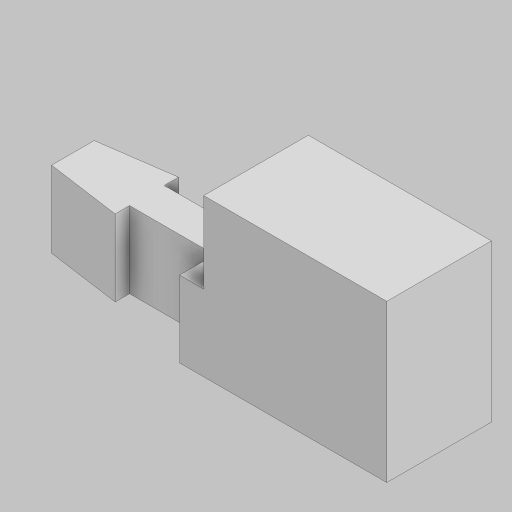
# Autodesk Inventor part: Tenon_Macho_Parametrizado
Saved by Autodesk Inventor 2023 (Build 270158000, 158)
## iProperties
Created: 2026-02-15
Part Number: Tenon_Macho_Parametrizado
Material: Genérico
Document SubType Name: Modeling
Designer: MARTIN MAESTRE
Density: 1 g/cm^3
Appearance: Valor por defecto
Author: MARTIN MAESTRE
Autodesk Inventor part; units mm, degrees
ref_plane "YZ Plane" through (0, 0, 0) normal (1, 0, 0) x (0, 1, 0)
ref_plane "XZ Plane" through (0, 0, 0) normal (0, 1, 0) x (-1, 0, 0)
ref_plane "XY Plane" through (0, 0, 0) normal (0, 0, 1) x (1, 0, 0)
sketch "Boceto1" plane through (0, 0, 0) normal (0, 0, 1) x (1, 0, 0)
  line L0 (0, 0) -> (28, 0)
  line L1 (28, 0) -> (28, 12)
  line L2 (28, 12) -> (0, 12)
  line L3 (0, 12) -> (0, 0)
  dimension "d0" = 28
  dimension "d1" = 12
  constraints: 8 end point, 3 perpendicular, 1 horizontal
  measures "d0" distance of L0.start L0.end
  measures "d1" distance of L0.end L1.end
extrude "Extrusión1" add sketch "Boceto1" along normal blind 8
sketch "Boceto2" plane through (0, 12, 0) normal (0, 1, 0) x (1, 0, 0)
  line L0 (28, -8) -> (0, -8) projected
  line L1 (0, 0) -> (0, -8)
  line L2 (28, 0) -> (0, 0) projected
  line L3 (0, 0) -> (14, 0)
  line L4 (0, 0) -> (14, 0) construction
  line L5 (14, 0) -> (14, -8)
  line L6 (0, -8) -> (14, -8)
  point P0 (14, 0)
  dimension "d4" = 14
  dimension "d5" = 0
  constraints: 10 end point, 3 collinear, 1 horizontal, 1 midpoint, 1 vertical
  measures "d4" distance of L1.start L3.end
  measures "d5" distance between parallel lines of L3 L4
extrude "Extrusión2" cut sketch "Boceto2" against normal blind 6.17
sketch "Boceto3" plane through (0, 0, 0) normal (0, -1, 0) x (1, 0, 0)
  line L0 (0, 0) -> (28, 0) projected
  line L1 (0, 0) -> (0, 2.37)
  line L2 (0, 0) -> (0, 8) projected
  line L3 (0, 2.37) -> (0, 5.63) construction
  line L4 (0, 5.63) -> (0, 8)
  line L5 (0, 0) -> (5.66, 0)
  line L6 (5.66, 0) -> (5.66, 1.57) construction
  line L7 (0, 2.37) -> (5.66, 1.57)
  line L8 (5.66, 0) -> (5.66, 1.57)
  line L9 (5.66, 1.57) -> (5.66, 2.67)
  line L10 (5.66, 2.67) -> (12.17, 2.67)
  line L11 (5.66, 0) -> (12.17, 0)
  line L12 (12.17, 0) -> (12.17, 2.67)
  line L13 (0, 8) -> (28, 8) projected
  line L14 (0, 8) -> (12.17, 8)
  line L15 (12.17, 8) -> (12.17, 5.33)
  line L16 (12.17, 5.33) -> (5.66, 5.33)
  line L17 (12.17, 5.33) -> (18.68, 5.33) construction
  line L18 (5.66, 5.33) -> (5.66, 6.43)
  line L19 (5.66, 6.43) -> (0, 5.63)
  dimension "d8" = 2.37
  dimension "d9" = 3.26
  dimension "d10" = 5.66
  dimension "d11" = 1.57
  dimension "d12" = 1.1
  dimension "d13" = 6.51
  dimension "d14" = 2.67
  dimension "d15" = 12.17
  dimension "d16" = 6.51
  dimension "d17" = 180
  dimension "d18" = 1.1
  constraints: 34 end point, 5 point on line, 4 perpendicular, 3 vertical, 2 collinear, 2 horizontal
  measures "d8" distance of L0.start L1.end
  measures "d9" distance of L1.end L3.end
  measures "d10" distance of L0.start L5.end
  measures "d11" distance of L5.end L6.end
  measures "d12" distance of L6.end L9.end
  measures "d13" distance of L9.end L10.end
  measures "d14" distance of L14.end L15.end
  measures "d15" distance between parallel lines of L2 L15
  measures "d16" distance of L15.end L16.end
  measures "d17" angle of L16 L17
  measures "d18" distance of L16.end L18.end
extrude "Extrusión3" cut sketch "Boceto3" against normal blind 6
equation "\"d4\" = Largo_mitad"
equation "\"d12\" = Prof_corte"
equation "\"d18\" = Prof_corte"
equation "\"Largo_mitad\" = 14"
equation "\"Prof_corte\" = 1.1"
equation "\"Separacion_1\" = 2.2"
equation "\"Separacion_2\" = 1.4"
equation "\"Separacion_3\" = 2.5"
equation "\"Angulo_0\" = 0"
equation "\"Angulo_180\" = 180deg"
